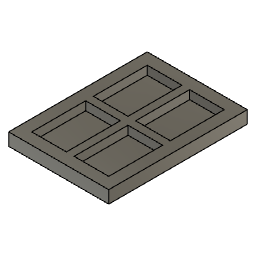
boardWindow (Autodesk Fusion 360 design; units mm, degrees)
Autodesk Fusion 360 part; units mm, degrees
sketch "Sketch1" plane through (0, 0, 0) normal (0, 0, 1) x (1, 0, 0)
  line L0 (0, 0) -> (26, 0)
  line L1 (26, 0) -> (26, 36)
  line L2 (26, 36) -> (0, 36)
  line L3 (0, 36) -> (0, 0)
  line L4 (3, 3) -> (23, 3)
  line L5 (3, 33) -> (3, 3)
  line L6 (23, 3) -> (23, 33)
  line L7 (23, 33) -> (3, 33)
  dimension "d2" = 30
  constraint horizontal L0
  constraint vertical L1
  constraint horizontal L2
  constraint vertical L3
  constraint horizontal L4
  constraint vertical L6
  constraint horizontal L7
  constraint vertical L5
  measures "d2" distance of L5.start L4.start
sketch "Sketch3" plane through (0, 0, 0) normal (0, 0, 1) x (1, 0, 0)
  line L0 (12, 33) -> (14, 33)
  line L1 (14, 33) -> (14, 3)
  line L2 (14, 3) -> (12, 3)
  line L3 (12, 3) -> (12, 33)
  line L4 (23, 19) -> (3, 19)
  line L5 (3, 19) -> (3, 17)
  line L6 (3, 17) -> (23, 17)
  line L7 (23, 17) -> (23, 19)
  constraint horizontal L0
  constraint vertical L1
  constraint horizontal L2
  constraint vertical L3
  constraint horizontal L4
  constraint vertical L5
  constraint horizontal L6
  constraint vertical L7
extrude "Extrude1" add sketch "Sketch1" along normal blind 4
extrude "Extrude5" add sketch "Sketch3" along normal blind 4 contours L0 L1 L3 L4 | L1 L3 L4 L6 | L1 L2 L3 L6
extrude "Extrude6" add sketch "Sketch3" along normal blind 4 contours L3 L4 L5 L6
extrude "Extrude7" add sketch "Sketch3" along normal blind 4 contours L1 L4 L6 L7
sketch "Sketch5" plane through (0, 0, 0) normal (0, 0, 1) x (1, 0, 0)
  line L0 (26, 36) -> (0, 36)
  line L1 (0, 0) -> (26, 0)
  line L2 (0, 36) -> (0, 0)
  line L3 (26, 0) -> (26, 36)
  constraint horizontal L1
  constraint vertical L3
  constraint horizontal L0
  constraint vertical L2
extrude "Extrude9" add sketch "Sketch5" along normal blind 1
sketch "Sketch6" plane through (0, 0, 4) normal (0, 0, 1) x (-1, 0, 0)
  line L0 (-14, -19) -> (-14, -33)
  line L1 (-14, -33) -> (-23, -33)
  line L2 (-23, -33) -> (-23, -19)
  line L3 (-23, -19) -> (-14, -19)
  line L4 (-3, -19) -> (-3, -33)
  line L5 (-3, -33) -> (-12, -33)
  line L6 (-12, -33) -> (-12, -19)
  line L7 (-12, -19) -> (-3, -19)
  line L8 (-14, -17) -> (-23, -17)
  line L9 (-23, -17) -> (-23, -3)
  line L10 (-23, -3) -> (-14, -3)
  line L11 (-14, -3) -> (-14, -17)
  line L12 (-3, -17) -> (-12, -17)
  line L13 (-12, -17) -> (-12, -3)
  line L14 (-12, -3) -> (-3, -3)
  line L15 (-3, -3) -> (-3, -17)
  line L16 (0, -36) -> (0, 0)
  line L17 (0, 0) -> (-26, 0)
  line L18 (-26, 0) -> (-26, -36)
  line L19 (-26, -36) -> (0, -36)
extrude "Extrude10" cut sketch "Sketch6" against normal blind 0.75
extrude "Extrude8" [suppressed]
extrude "Extrude4" [suppressed]
extrude "Extrude3" [suppressed]
extrude "Extrude2" [suppressed]
